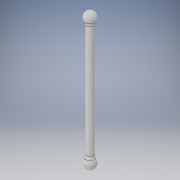
# Autodesk Inventor part: Component 39(Rod)
Saved by Autodesk Inventor 2018 (Build 220112000, 112)
## iProperties
Created: 2023-04-01
Part Number: Component 39(Rod)
Material: Generic
Document SubType Name: Modeling
Designer: Habib Mohamed
Density: 1 g/cm^3
Appearance: Default
Author: Habib Mohamed
Autodesk Inventor part; units mm, degrees
ref_plane "YZ Plane" through (0, 0, 0) normal (1, 0, 0) x (0, 1, 0)
ref_plane "XZ Plane" through (0, 0, 0) normal (0, 1, 0) x (-1, 0, 0)
ref_plane "XY Plane" through (0, 0, 0) normal (0, 0, 1) x (1, 0, 0)
sketch "Sketch1" plane through (0, 0, 0) normal (1, 0, 0) x (0, 1, 0)
  arc A0 (24.1787, -1.9444) -> (28.25, 0) centre (25.75, 0) ccw
  line L0 (25.75, 0) -> (0, 0)
  line L1 (22.9216, -1.5) -> (0, -1.5)
  line L2 (28.25, 0) -> (25.75, 0)
  arc A1 (24.1787, -1.9444) -> (22.9216, -1.5) centre (22.9216, -3.5) ccw
  line L3 (0, 0) -> (0, -7.7496) construction
  arc A2 (-28.25, 0) -> (-24.1787, -1.9444) centre (-25.75, 0) ccw
  line L4 (-25.75, 0) -> (0, 0)
  line L5 (-22.9216, -1.5) -> (0, -1.5)
  line L6 (-28.25, 0) -> (-25.75, 0)
  arc A3 (-22.9216, -1.5) -> (-24.1787, -1.9444) centre (-22.9216, -3.5) ccw
  point P0 (23.75, -1.5)
  point P1 (-23.75, -1.5)
  dimension "d0" = 5
  dimension "d1" = 1.5
  dimension "d2" = 25.75
  dimension "d3" = 2
  constraints: 14 end point, 10 point on circle, 6 symmetric about line, 4 centre point, 3 horizontal, 2 point on line, 2 tangent, 1 vertical, 2 other
  measures "d0" diameter of A0
  measures "d1" distance between parallel lines of L1 L0
  measures "d2" distance of L0.start L0.end
  measures "d3" radius of A1
revolve "Revolution1" add sketch "Sketch1" angle 360 about axis through (0, 25.75, 0) along (0, -1, 0)
body "Solid1"
